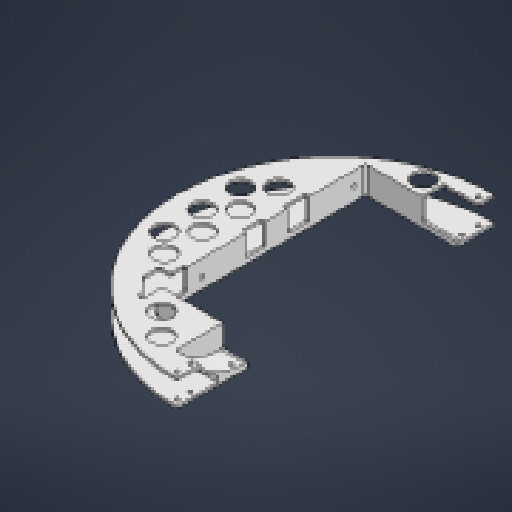
# Autodesk Inventor part: 3DPRINT,CABLE-SHROUD
Saved by Autodesk Inventor 2026 (Build 300175000, 175)
## iProperties
Created: 2026-02-11
Part Number: 3DPRINT,CABLE-SHROUD
Material: Generic
Document SubType Name: Modeling
Designer: littl
Density: 1 g/cm^3
Appearance: Default
Author: littl
Autodesk Inventor part; units mm, degrees
ref_plane "YZ Plane" through (0, 0, 0) normal (1, 0, 0) x (0, 1, 0)
ref_plane "XZ Plane" through (0, 0, 0) normal (0, 1, 0) x (-1, 0, 0)
ref_plane "XY Plane" through (0, 0, 0) normal (0, 0, 1) x (1, 0, 0)
sketch "Sketch1" plane through (0, 0, 0) normal (0, 1, 0) x (-1, 0, 0)
  circle A0 centre (0, 0) radius 185.7375
  line L0 (103.1875, 102.832154) -> (-103.1875, 102.832154)
  line L1 (-106.3625, 99.657154) -> (-106.3625, -138.467846)
  line L2 (-103.1875, -141.642846) -> (103.1875, -141.642846)
  line L3 (106.3625, -138.467846) -> (106.3625, 99.657154)
  line L4 (106.3625, 102.832154) -> (-106.3625, -141.642846) construction
  line L5 (-106.3625, 102.832154) -> (106.3625, -141.642846) construction
  arc A1 (106.3625, 99.657154) -> (103.1875, 102.832154) centre (103.1875, 99.657154) ccw
  arc A2 (-103.1875, 102.832154) -> (-106.3625, 99.657154) centre (-103.1875, 99.657154) ccw
  arc A3 (-106.3625, -138.467846) -> (-103.1875, -141.642846) centre (-103.1875, -138.467846) ccw
  arc A4 (103.1875, -141.642846) -> (106.3625, -138.467846) centre (103.1875, -138.467846) ccw
  point P0 (0, -19.405346)
  dimension "d0" = 371.475
  dimension "d1" = 102.83215
  dimension "d2" = 244.475
  dimension "d3" = 212.725
  dimension "d6" = 3.175
  constraints: 12 end point, 8 point on circle, 8 point on line, 8 tangent, 5 centre point, 3 equal radius, 2 midpoint, 2 parallel, 1 coincident, 1 horizontal, 1 perpendicular, 1 vertical alignment
  measures "d0" diameter of A0
  measures "d1" distance from line of point (0, 0) L0
  measures "d2" distance of L5.end L4.start
  measures "d3" distance of L4.end L5.end
  measures "d6" radius of A1
extrude "Extrusion1" add sketch "Sketch1" along normal blind 3.175
sketch "Sketch2" plane through (0, 3.175, 0) normal (0, 1, 0) x (1, 0, 0)
  circle A0 centre (0, 0) radius 185.7375
  arc A1 (-106.3625, -99.657154) -> (-103.1875, -102.832154) centre (-103.1875, -99.657154) ccw
  line L0 (-106.3625, -99.657154) -> (-106.3625, 138.467846)
  arc A2 (-103.1875, 141.642846) -> (-106.3625, 138.467846) centre (-103.1875, 138.467846) ccw
  line L1 (-103.1875, 141.642846) -> (103.1875, 141.642846)
  arc A3 (106.3625, 138.467846) -> (103.1875, 141.642846) centre (103.1875, 138.467846) ccw
  line L2 (106.3625, 138.467846) -> (106.3625, -99.657154)
  arc A4 (103.1875, -102.832154) -> (106.3625, -99.657154) centre (103.1875, -99.657154) ccw
  line L3 (103.1875, -102.832154) -> (-103.1875, -102.832154)
  line L4 (103.1875, 144.817846) -> (-103.1875, 144.817846)
  arc A5 (-103.1875, 144.817846) -> (-109.5375, 138.467846) centre (-103.1875, 138.467846) ccw
  line L5 (-109.5375, 138.467846) -> (-109.5375, -99.657154)
  arc A6 (-109.5375, -99.657154) -> (-103.1875, -106.007154) centre (-103.1875, -99.657154) ccw
  line L6 (-103.1875, -106.007154) -> (103.1875, -106.007154)
  arc A7 (103.1875, -106.007154) -> (109.5375, -99.657154) centre (103.1875, -99.657154) ccw
  line L7 (109.5375, -99.657154) -> (109.5375, 138.467846)
  arc A8 (109.5375, 138.467846) -> (103.1875, 144.817846) centre (103.1875, 138.467846) ccw
  dimension "d7" = 3.175
  constraints: 8 end point, 8 point on circle, 4 centre point, 7 other
  measures "d7" distance between parallel lines of L1 L4
extrude "Extrusion2" add sketch "Sketch2" along normal blind 12.7 contours A8 L7 A7 L6 A6 L5 A5 L4
mirror "Mirror2" about plane through (0, 15.875, -19.405346) normal (0, 1, 0) of "Extrusion1", "Extrusion2"
sketch "Sketch3" plane through (0, 31.75, 0) normal (0, 1, 0) x (1, 0, 0)
  line L0 (-106.3625, -99.657154) -> (-106.3625, 138.467846)
  line L1 (-106.3625, -67.907154) -> (-109.5375, -67.907154)
  line L2 (-109.5375, -67.907154) -> (-109.5375, -93.307154)
  line L3 (-109.5375, -93.307154) -> (-106.3625, -93.307154)
  line L4 (-106.3625, -93.307154) -> (-106.3625, -67.907154)
  line L5 (-106.3625, 24.167846) -> (-111.4425, 24.167846)
  line L6 (-111.4425, 24.167846) -> (-111.4425, 1.942846)
  line L7 (-111.4425, 1.942846) -> (-106.3625, 1.942846)
  line L8 (-106.3625, 1.942846) -> (-106.3625, 24.167846)
  line L9 (-106.3625, 50.202846) -> (-111.4425, 50.202846)
  line L10 (-111.4425, 50.202846) -> (-111.4425, 75.602846)
  line L11 (-111.4425, 75.602846) -> (-106.3625, 75.602846)
  line L12 (-106.3625, 75.602846) -> (-106.3625, 50.202846)
  line L13 (-103.1875, 141.642846) -> (103.1875, 141.642846)
  line L14 (40.64, 141.642846) -> (-40.64, 141.642846)
  line L15 (-40.64, 141.642846) -> (-40.64, 167.042846)
  line L16 (-40.64, 167.042846) -> (40.64, 167.042846)
  line L17 (40.64, 167.042846) -> (40.64, 141.642846)
  arc A0 (-106.3625, -99.657154) -> (-103.1875, -102.832154) centre (-103.1875, -99.657154) ccw
  line L18 (-106.3625, -99.657154) -> (-100.0125, -99.657154)
  line L19 (-100.0125, -99.657154) -> (-100.0125, -125.057154)
  line L20 (-100.0125, -125.057154) -> (-106.3625, -125.057154)
  line L21 (-106.3625, -125.057154) -> (-106.3625, -99.657154)
  line L22 (103.1875, -102.832154) -> (-103.1875, -102.832154)
  line L23 (-28.575, -102.832154) -> (28.575, -102.832154)
  line L24 (28.575, -102.832154) -> (28.575, -158.394654)
  line L25 (28.575, -158.394654) -> (-28.575, -158.394654)
  line L26 (-28.575, -158.394654) -> (-28.575, -102.832154)
  line L27 (-106.3625, -102.832154) -> (-122.2375, -102.832154)
  line L28 (-122.2375, -102.832154) -> (-122.2375, -83.782154)
  line L29 (-122.2375, -83.782154) -> (-106.3625, -83.782154)
  line L30 (-106.3625, -83.782154) -> (-106.3625, -102.832154)
  line L31 (-122.2375, -102.832154) -> (-106.3625, -118.707154)
  line L32 (-122.2375, -102.832154) -> (-99.78686, -102.832154) construction
  line L33 (0, -102.832154) -> (0, 141.642846) construction
  line L34 (106.3625, -67.907154) -> (109.5375, -67.907154)
  line L35 (109.5375, -67.907154) -> (109.5375, -93.307154)
  line L36 (109.5375, -93.307154) -> (106.3625, -93.307154)
  line L37 (106.3625, -93.307154) -> (106.3625, -67.907154)
  line L38 (106.3625, 24.167846) -> (111.4425, 24.167846)
  line L39 (111.4425, 24.167846) -> (111.4425, 1.942846)
  line L40 (111.4425, 1.942846) -> (106.3625, 1.942846)
  line L41 (106.3625, 1.942846) -> (106.3625, 24.167846)
  line L42 (106.3625, 50.202846) -> (111.4425, 50.202846)
  line L43 (111.4425, 50.202846) -> (111.4425, 75.602846)
  line L44 (111.4425, 75.602846) -> (106.3625, 75.602846)
  line L45 (106.3625, 75.602846) -> (106.3625, 50.202846)
  line L46 (106.3625, -99.657154) -> (100.0125, -99.657154)
  line L47 (100.0125, -99.657154) -> (100.0125, -125.057154)
  line L48 (100.0125, -125.057154) -> (106.3625, -125.057154)
  line L49 (106.3625, -125.057154) -> (106.3625, -99.657154)
  line L50 (106.3625, -67.907154) -> (109.5375, -67.907154)
  line L51 (109.5375, -67.907154) -> (109.5375, -93.307154)
  line L52 (109.5375, -93.307154) -> (106.3625, -93.307154)
  line L53 (106.3625, -93.307154) -> (106.3625, -67.907154)
  line L54 (106.3625, 24.167846) -> (111.4425, 24.167846)
  line L55 (111.4425, 24.167846) -> (111.4425, 1.942846)
  line L56 (111.4425, 1.942846) -> (106.3625, 1.942846)
  line L57 (106.3625, 1.942846) -> (106.3625, 24.167846)
  line L58 (106.3625, 50.202846) -> (111.4425, 50.202846)
  line L59 (111.4425, 50.202846) -> (111.4425, 75.602846)
  line L60 (111.4425, 75.602846) -> (106.3625, 75.602846)
  line L61 (106.3625, 75.602846) -> (106.3625, 50.202846)
  arc A1 (103.1875, -102.832154) -> (106.3625, -99.657154) centre (103.1875, -99.657154) ccw
  line L62 (106.3625, -99.657154) -> (100.0125, -99.657154)
  line L63 (100.0125, -99.657154) -> (100.0125, -125.057154)
  line L64 (100.0125, -125.057154) -> (106.3625, -125.057154)
  line L65 (106.3625, -125.057154) -> (106.3625, -99.657154)
  line L66 (106.3625, -102.832154) -> (122.2375, -102.832154)
  line L67 (122.2375, -102.832154) -> (122.2375, -83.782154)
  line L68 (122.2375, -83.782154) -> (106.3625, -83.782154)
  line L69 (106.3625, -83.782154) -> (106.3625, -102.832154)
  line L70 (122.2375, -102.832154) -> (106.3625, -118.707154)
  line L71 (122.2375, -102.832154) -> (99.78686, -102.832154) construction
  point P0 (0, 0)
  point P1 (0, 167.042846)
  point P2 (0, -158.394654)
  point P3 (-100.0125, -102.832154)
  point P4 (-109.5375, -83.782154)
  point P5 (109.5375, -83.782154)
  dimension "d13" = 3.175
  dimension "d14" = 25.4
  dimension "d15" = 6.35
  dimension "d16" = 25.4
  dimension "d17" = 57.15
  dimension "d18" = 55.5625
  dimension "d19" = 9.525
  dimension "d20" = 25.4
  dimension "d21" = 22.225
  dimension "d22" = 104.775
  dimension "d23" = 5.08
  dimension "d24" = 66.04
  dimension "d25" = 81.28
  dimension "d28" = 15.875
  dimension "d29" = 19.05
  dimension "d30" = 45
  constraints: 138 end point, 23 symmetric about line, 14 parallel, 12 point on line, 8 horizontal, 8 perpendicular, 4 midpoint, 2 equal length, 2 point on circle, 2 vertical alignment, 1 centre point, 1 collinear, 1 other
  measures "d13" distance of L3.end L2.end
  measures "d14" distance of L14.end L15.end
  measures "d15" distance of L19.end L20.end
  measures "d16" distance of L18.end L19.end
  measures "d17" distance of L24.end L25.end
  measures "d18" distance between parallel lines of L23 L25
  measures "d19" distance between parallel lines of L22 L3
  measures "d20" distance between parallel lines of L3 L1
  measures "d21" distance of L5.end L6.end
  measures "d22" distance between parallel lines of L22 L7
  measures "d23" distance between parallel lines of L8 L6
  measures "d24" distance between parallel lines of L13 L11
  measures "d25" distance of L15.end L16.end
  measures "d28" distance of L28.end L29.end
  measures "d29" distance of L27.end L28.end
  measures "d30" angle of L31 L32
extrude "Extrusion3" cut sketch "Sketch3" against normal blind 25.4 contours L21 L27 L28 L29 L2 L3 L0 | A0 L22 L19 L20 L21 | L3 L2 L29 L0 | L21 L31 L27 | L29 L2 L1 L0 | L7 L6 L5 L0 | L9 L10 L11 L0 | L15 L16 L17 L13 | L24 L25 L26 L22 | A1 L49 L48 L47 L22 | L22 L47 L46 A1 | L69 L36 L35 L68 L67 L66 L49 | L66 L70 L49 | L37 L68 L35 L36 | L37 L34 L35 L68 | L38 L39 L40 L41 | L45 L44 L43 L42
fillet "Fillet1" radius 1.5875 42 edges at (-122.2375, 30.1625, 83.7822) (-122.2375, 30.1625, 102.8322) (-106.3625, 30.1625, 118.7072) (-100.0125, 30.1625, 125.0572) (-106.3625, 30.1625, 125.0572) (-28.575, 30.1625, 158.3947) (28.575, 30.1625, 158.3947) (-111.4425, 30.1625, -1.9428) (-111.4425, 30.1625, -24.1678) (-111.4425, 30.1625, -50.2028) (-111.4425, 30.1625, -75.6028) (-40.64, 30.1625, -167.0428) (40.64, 30.1625, -167.0428) (-109.5375, 30.1625, 83.7822) (-109.5375, 30.1625, 67.9072) (-107.95, 6.35, -50.2028) (-107.95, 6.35, -75.6028) (-107.95, 6.35, -24.1678) (-107.95, 6.35, -1.9428) (-107.95, 6.35, 67.9072) (-100.0125, 6.35, 104.4197) (-28.575, 6.35, 104.4197) (28.575, 6.35, 104.4197) (40.64, 6.35, -143.2303) (-40.64, 6.35, -143.2303) (100.0125, 30.1625, 125.0572) (106.3625, 30.1625, 125.0572) (106.3625, 30.1625, 118.7072) (122.2375, 30.1625, 102.8322) (122.2375, 30.1625, 83.7822) (109.5375, 30.1625, 83.7822) (109.5375, 30.1625, 67.9072) (100.0125, 6.35, 104.4197) (107.95, 6.35, 67.9072) (111.4425, 30.1625, -1.9428) (111.4425, 30.1625, -24.1678) (111.4425, 30.1625, -75.6028) (111.4425, 30.1625, -50.2028) (107.95, 6.35, -50.2028) (107.95, 6.35, -75.6028) (107.95, 6.35, -1.9428) (107.95, 6.35, -24.1678)
sketch "Sketch4" plane through (-106.3625, 0, 99.657154) normal (1, 0, 0) x (0, 0, -1)
  line L0 (0, 3.175) -> (238.125, 3.175) projected
  line L1 (175.26, 7.9375) -> (175.26, 28.575) projected
  line L2 (31.75, 7.9375) -> (31.75, 28.575) projected
  point P0 (99.657154, 0)
  point P1 (49.87292, 12.7)
  point P2 (227.67292, 15.875)
  dimension "d32" = 12.7
  dimension "d33" = 9.525
  dimension "d34" = 52.41292
  dimension "d35" = 18.12292
  measures "d32" distance from line of L0 point (227.673, 15.875)
  measures "d33" distance from line of L0 point (49.873, 12.7)
  measures "d34" distance from line of L1 point (227.673, 15.875)
  measures "d35" distance from line of L2 point (49.873, 12.7)
hole "Hole1" at (-106.3625, 12.7, 49.784234) at (-106.3625, 15.875, -128.015766) direction (-1, 0, 0) diameter 4.9784 end through all clearance for "Flat Head Machine Screw (82)" size "#10" standard "Ansi Unified Screw Threads"
mirror "Mirror3" about plane through (0, 0, 0) normal (1, 0, 0) of "Hole1"
sketch "Sketch5" plane through (0, 0, 0) normal (1, 0, 0) x (0, 1, 0)
  line L0 (6.35, 102.832154) -> (6.35, 106.007154)
  line L1 (28.575, 158.394654) -> (31.75, 158.394654)
  arc A0 (28.575, 158.394654) -> (6.35, 106.007154) centre (79.204911, 106.007154) ccw
  line L2 (6.35, 106.007154) -> (3.175, 106.007154)
  line L3 (28.575, 106.007154) -> (7.9375, 106.007154)
  line L4 (6.35, 106.007154) -> (7.9375, 106.007154)
  line L5 (3.175, 106.007154) -> (6.35, 106.007154)
  line L6 (3.175, 106.007154) -> (6.35, 106.007154)
  line L7 (7.9375, 106.007154) -> (6.35, 106.007154)
  line L8 (7.9375, 106.007154) -> (28.575, 106.007154)
  line L9 (28.575, 106.007154) -> (7.9375, 106.007154)
  line L10 (6.35, 106.007154) -> (7.9375, 106.007154)
  line L11 (7.9375, 106.007154) -> (6.35, 106.007154)
  line L12 (7.9375, 106.007154) -> (28.575, 106.007154)
  arc A1 (28.575, 161.569654) -> (3.175, 106.007154) centre (76.646484, 106.007154) ccw
  line L13 (28.575, 158.394654) -> (28.575, 161.569654)
  line L14 (10.389436, 137.757154) -> (3.175, 137.757154)
  line L15 (3.175, 137.757154) -> (3.175, 106.007154)
  line L16 (3.175, -185.7375) -> (3.175, 185.7375)
  point P0 (0, 0)
  dimension "d43" = 3.175
  dimension "d44" = 3.175
  dimension "d45" = 0
  dimension "d50" = 31.75
  constraints: 8 end point, 6 point on circle, 2 centre point, 2 collinear, 2 horizontal, 1 tangent, 1 vertical
  measures "d43" distance of L2.start L2.end
  measures "d44" distance of L1.start L13.end
  measures "d45" vertical distance of A1.centre A0.centre
  measures "d50" distance between parallel lines of L6 L14
extrude "Extrusion4" add sketch "Sketch5" along normal mid plane 57.15
sketch "Sketch7" plane through (-28.575, 0, 0) normal (-1, 0, 0) x (0, 0, 1)
  arc A0 (137.757154, 10.389436) -> (161.569654, 28.575) centre (106.007154, 76.646484) ccw
  line L0 (137.757154, 3.175) -> (137.757154, 10.389436)
  line L1 (137.757154, 3.175) -> (106.007154, 3.175)
  line L2 (106.007154, 7.9375) -> (106.007154, 28.575)
  line L3 (106.007154, 3.175) -> (106.007154, 28.575)
  line L4 (106.007154, 28.575) -> (161.569654, 28.575)
  point P0 (0, 0)
  constraints: 4 end point, 1 collinear, 1 perpendicular
extrude "Extrusion6" add sketch "Sketch7" along normal blind 3.175
mirror "Mirror4" about plane through (0, 0, 0) normal (1, 0, 0) of "Extrusion6"
fillet "Fillet2" radius 1.5875 7 edges at (-31.75, 18.2555, 150.6003) (-31.75, 6.7822, 137.7572) (31.75, 6.7822, 137.7572) (31.75, 18.2555, 150.6003) (0, 10.3894, 137.7572) (-31.75, 3.175, 121.8822) (31.75, 3.175, 121.8822)
sketch "Sketch8" plane through (0, 0, 0) normal (1, 0, 0) x (0, 1, 0)
  line L0 (31.75, -185.7375) -> (31.75, 185.7375) projected
  line L1 (0, -185.7375) -> (0, 185.7375) projected
  line L2 (31.75, -185.7375) -> (0, -185.7375)
  line L3 (0, -185.7375) -> (0, 185.7375)
  line L4 (0, 185.7375) -> (31.75, 185.7375)
  line L5 (31.75, 185.7375) -> (31.75, -185.7375)
  point P0 (0, 0)
  constraints: 8 end point, 2 parallel, 1 horizontal, 1 perpendicular
extrude "Extrusion7" cut sketch "Sketch8" along normal blind 190.5
sketch "Sketch9" plane through (0, 3.175, 0) normal (0, 1, 0) x (1, 0, 0)
  line L0 (-103.1875, 141.642846) -> (0, 141.642846)
  line L1 (0, 185.7375) -> (0, 141.642846)
  point P0 (0, 0)
  point P1 (-6.35, 154.342846)
  point P2 (-6.35, 173.392846)
  dimension "d57" = 19.05
  dimension "d58" = 12.7
  dimension "d59" = 6.35
  constraints: 1 vertical alignment
  measures "d57" distance of point (-6.35, 154.343) point (-6.35, 173.393)
  measures "d58" distance from line of L0 point (-6.35, 154.343)
  measures "d59" distance from line of L1 point (-6.35, 173.393)
hole "Hole2" at (-6.35, 3.175, -154.342846) at (-6.35, 3.175, -173.392846) direction (0, -1, 0) diameter 5.08 end through all both
sketch "Sketch10" plane through (0, 3.175, 0) normal (0, 1, 0) x (1, 0, 0)
  line L0 (0, -102.832154) -> (-103.1875, -102.832154)
  line L1 (0, -102.832154) -> (0, -185.7375)
  point P0 (0, 0)
  point P1 (-6.35, -115.532154)
  point P2 (-6.35, -179.032154)
  point P3 (-6.35, -163.157154)
  dimension "d67" = 63.5
  dimension "d68" = 12.7
  dimension "d69" = 15.875
  dimension "d70" = 6.35
  constraints: 2 vertical alignment
  measures "d67" distance of point (-6.35, -179.032) point (-6.35, -115.532)
  measures "d68" distance from line of L0 point (-6.35, -115.532)
  measures "d69" distance of point (-6.35, -179.032) point (-6.35, -163.157)
  measures "d70" distance from line of L1 point (-6.35, -179.032)
hole "Hole3" at (-6.35, 3.175, 115.532154) at (-6.35, 3.175, 179.032154) at (-6.35, 3.175, 163.157154) direction (0, -1, 0) diameter 5.08 end through all both
sketch "Sketch11" plane through (-100.0125, 31.75, 102.832154) normal (0, 1, 0) x (1, 0, 0)
  circle A0 centre (-55.5625, 169.507154) radius 12.7
  line L0 (100.0125, 362.864654) -> (100.0125, -157.200346) construction
  line L1 (-123.435678, 102.832154) -> (137.253863, 102.832154) construction
  circle A1 centre (-33.3375, 169.507154) radius 12.7
  circle A2 centre (-55.5625, 147.282154) radius 12.7
  circle A3 centre (-33.3375, 147.282154) radius 12.7
  circle A4 centre (-55.5625, 125.057154) radius 12.7
  circle A5 centre (-33.3375, 125.057154) radius 12.7
  circle A6 centre (-55.5625, 102.832154) radius 12.7
  circle A7 centre (-33.3375, 102.832154) radius 12.7
  circle A8 centre (-55.5625, 80.607154) radius 12.7
  circle A9 centre (-33.3375, 80.607154) radius 12.7
  circle A10 centre (-55.5625, 58.382154) radius 12.7
  circle A11 centre (-33.3375, 58.382154) radius 12.7
  circle A12 centre (-55.5625, 36.157154) radius 12.7
  circle A13 centre (-33.3375, 36.157154) radius 12.7
  circle A14 centre (49.2125, -49.567846) radius 12.7
  circle A15 centre (42.8625, 262.852154) radius 12.7
  circle A16 centre (23.8125, -24.167846) radius 12.7
  point P0 (100.0125, 102.832154)
  dimension "d78" = 25.4
  dimension "d81" = 22.225
  dimension "d84" = 22.225
  dimension "d87" = 155.575
  dimension "d90" = 127
  dimension "d91" = 76.2
  dimension "d92" = 152.4
  dimension "d93" = 50.8
  dimension "d94" = 57.15
  dimension "d95" = 160.02
  constraints: 17 centre point, 3 equal radius, 1 horizontal, 1 horizontal alignment, 1 vertical, 26 other
  measures "d78" diameter of A0
  measures "d81" distance of A0.centre A1.centre
  measures "d84" distance of A0.centre A2.centre
  measures "d87" distance of point (100.012, 102.832) A6.centre
  measures "d90" distance from line of L1 A16.centre
  measures "d91" distance from line of L0 A16.centre
  measures "d92" distance from line of L1 A14.centre
  measures "d93" distance from line of L0 A14.centre
  measures "d94" distance from line of L0 A15.centre
  measures "d95" distance from line of L1 A15.centre
extrude "Extrusion8" cut sketch "Sketch11" against normal up to surface (3.175 mm away) contours A0 A1 | A0 A1 A3 | A2 A0 | A0 A2 A3 A4 | A3 A1 | A4 A2 | A2 A3 | A6 A4 | A4 A6 A7 A8 | A5 A3 A7 A4 | A4 A5 | A8 A6 | A3 A5 | A6 A7 | A10 A8 | A8 A10 A11 A12 | A7 A5 | A9 A7 A11 A8 | A8 A9 | A12 A10 | A9 A7 | A10 A11 | A13 A12 | A12 A13 A11 | A11 A9 | A13 A11 | A14 | A15 | A16
body "Solid1"
